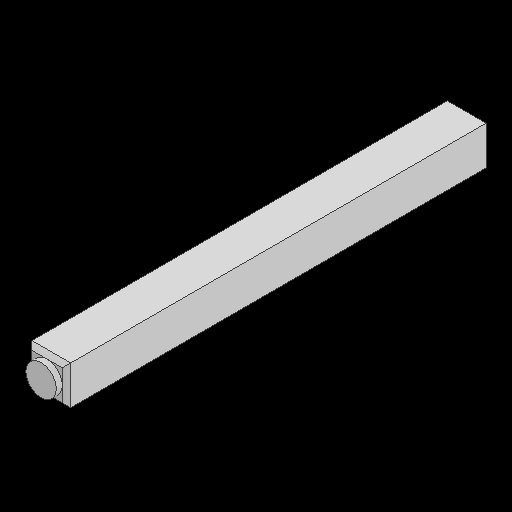
# Autodesk Inventor part: Pin_7mm
Saved by Autodesk Inventor 2027.1 (Build 311270010, 270A)
## iProperties
Created: 2026-10-09
Part Number: Pin_7mm
Material: Generisch
Document SubType Name: Modeling
Designer: josia
Density: 1 g/cm^3
Appearance: Vorgabe
Author: josia
Autodesk Inventor part; units mm, degrees
ref_plane "YZ Plane" through (0, 0, 0) normal (1, 0, 0) x (0, 1, 0)
ref_plane "XZ Plane" through (0, 0, 0) normal (0, 1, 0) x (-1, 0, 0)
ref_plane "XY Plane" through (0, 0, 0) normal (0, 0, 1) x (1, 0, 0)
sketch "Skizze1" plane through (0, 0, 0) normal (0, 1, 0) x (-1, 0, 0)
  line L0 (-0.32, -3.5) -> (0.32, -3.5)
  line L1 (0.32, -3.5) -> (0.32, 3.5)
  line L2 (0.32, 3.5) -> (-0.32, 3.5)
  line L3 (-0.32, 3.5) -> (-0.32, -3.5)
  line L4 (-0.32, -3.5) -> (0.32, 3.5) construction
  line L5 (0.32, -3.5) -> (-0.32, 3.5) construction
  point P0 (0, 0)
  point P1 (0, -3.5)
  point P2 (0, 3.5)
  dimension "d0" = 0.64
  dimension "d1" = 7
  constraints: 12 end point, 4 midpoint, 2 parallel, 1 horizontal, 1 perpendicular
  measures "d0" distance of L2.end L1.end
  measures "d1" distance of point (0, -3.5) point (0, 3.5)
extrude "Extrusion1" add sketch "Skizze1" along normal blind 0.64
chamfer "Fasen1" distance 0.07 angle 45 8 edges at (0, 0.64, 3.5) (0.32, 0.32, 3.5) (-0.32, 0.32, 3.5) (0, 0, 3.5) (0.32, 0.32, -3.5) (0, 0.64, -3.5) (-0.32, 0.32, -3.5) (0, 0, -3.5)
sketch "Skizze2" plane through (-0.25, 0.07, 3.5) normal (0, 0, 1) x (1, 0, 0)
  line L0 (0, 0.5) -> (0, 0) projected
  line L1 (0, 0) -> (0.5, 0) projected
  line L2 (0, 0.5) -> (0.5, 0)
  line L3 (0.5, 0) -> (0.5, 0.5) projected
  line L4 (0.5, 0) -> (0.5, 0.5)
  line L5 (0.5, 0.5) -> (0, 0)
  circle A0 centre (0.25, 0.25) radius 0.25
  line L6 (0.5, 0.5) -> (0, 0.5) projected
  point P0 (0.25, -0.07)
  constraints: 6 end point, 1 centre point, 1 collinear, 1 midpoint, 1 perpendicular, 1 tangent
extrude "Extrusion2" add sketch "Skizze2" along normal blind 0.1 contours A0 L2 L5 | A0 L5 L2 | L5 L2 A0 | L5 A0 L2
